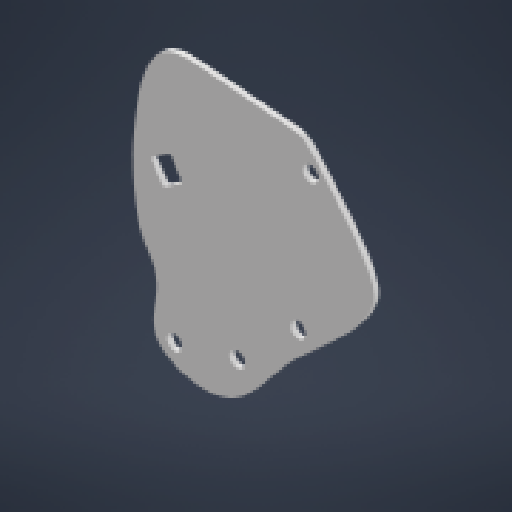
# Autodesk Inventor part: tracking-wheet-outer-mount-v2
Saved by Autodesk Inventor 2023.2 (Build 272271000, 271)
## iProperties
Created: 2023-04-12
Part Number: tracking-wheet-outer-mount-v2
Material: Generic
Document SubType Name: Modeling
Designer: Liam
Density: 1 g/cm^3
Appearance: Default
Author: Liam
Autodesk Inventor part; units mm, degrees
ref_plane "YZ Plane" through (0, 0, 0) normal (1, 0, 0) x (0, 1, 0)
ref_plane "XZ Plane" through (0, 0, 0) normal (0, 1, 0) x (-1, 0, 0)
ref_plane "XY Plane" through (0, 0, 0) normal (0, 0, 1) x (1, 0, 0)
sketch "Sketch1" plane through (0, 0, 0) normal (0, 0, 1) x (1, 0, 0)
  spline S0 degree 4 poles (36.0337, 7.5688) (36.414, 11.9825) (28.7931, 22.5974) (17.6153, 35.7287) (16.2127, 36.4244) (12.1158, 36.7774) (8.4963, 37.0893) (2.2009, 37.6317) (-1.6462, 37.9632) (-16.3236, 39.2278) (-18.5834, 39.4225) (-28.021, 34.4139) (-29.8449, 13.245) knots -10 -10 -10 -10 -10 -9 -8 -7 -6 -5 -4 -3 -2 -1 -1 -1 -1 -1 projected
  spline S1 degree 4 poles (-29.8449, 13.245) (-30.3855, 6.9715) (-29.3895, -8.4449) (-25.0846, -11.9416) (-21.5103, -19.5684) (-27.4136, -30.8853) (-16.5352, -37.6974) (-4.2729, -37.5026) (2.5545, -32.1215) (9.356, -22.2279) (17.0371, -15.0646) (23.4948, -9.4314) (30.8769, -2.7502) (35.7978, 4.8301) (36.0337, 7.5688) knots -12 -12 -12 -12 -12 -11 -10 -9 -8 -7 -6 -5 -4 -3 -2 -1 -1 -1 -1 -1 projected
  circle A0 centre (-1.3811, -25.4474) radius 2.0955 projected
  circle A1 centre (-18.6117, -30.0188) radius 2.0955 projected
  circle A2 centre (18.6969, 28.61) radius 2.0955 projected
  circle A3 centre (15.3532, -10.1968) radius 2.0955 projected
  arc A4 (-24.582, 10.9851) -> (-24.7636, 10.1056) centre (-24.233, 10.4545) ccw projected
  line L0 (-24.582, 10.9851) -> (-20.3376, 13.7765) projected
  arc A5 (-19.4581, 13.5949) -> (-20.3376, 13.7765) centre (-19.9887, 13.246) ccw projected
  line L1 (-19.4581, 13.5949) -> (-16.6667, 9.3506) projected
  arc A6 (-16.8484, 8.4711) -> (-16.6667, 9.3506) centre (-17.1973, 9.0016) ccw projected
  line L2 (-16.8484, 8.4711) -> (-21.0927, 5.6797) projected
  arc A7 (-21.9722, 5.8613) -> (-21.0927, 5.6797) centre (-21.4416, 6.2102) ccw projected
  line L3 (-21.9722, 5.8613) -> (-24.7636, 10.1056) projected
  circle A8 centre (4.6807, 9.27) radius 2.0955
  line L4 (-17.1973, 9.0016) -> (-24.233, 10.4545) construction
  point P0 (-20.7152, 9.7281)
  dimension "d9" = 4.191
  constraints: 2 end point, 1 centre point, 1 midpoint, 1 other
  measures "d9" diameter of A8
extrude "Extrusion1" add sketch "Sketch1" along normal blind 1.524
body "Solid1"
